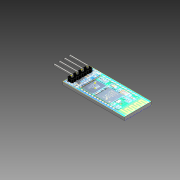
# Autodesk Inventor part: BLUTOOTH
Saved by Autodesk Inventor 2016 (Build 200138000, 138)
## iProperties
Created: 2017-05-25
Part Number: BLUTOOTH
Material: Generic
Document SubType Name: Modeling
Designer: USER
Density: 1 g/cm^3
Appearance: Default
Author: USER
Autodesk Inventor part; units mm, degrees
ref_plane "YZ Plane" through (0, 0, 0) normal (1, 0, 0) x (0, 1, 0)
ref_plane "XZ Plane" through (0, 0, 0) normal (0, 1, 0) x (-1, 0, 0)
ref_plane "XY Plane" through (0, 0, 0) normal (0, 0, 1) x (1, 0, 0)
sketch "Sketch1" plane through (0, 0, 0) normal (0, 0, 1) x (1, 0, 0)
  line L0 (-10.8819, 8.2952) -> (19.3441, 8.2952)
  line L1 (19.3441, 8.2952) -> (19.3441, -4.9318)
  line L2 (19.3441, -4.9318) -> (-10.8819, -4.9318)
  line L3 (-10.8819, -4.9318) -> (-10.8819, 8.2952)
  point P0 (0, 0)
  dimension "d0" = 30.226
  dimension "d1" = 13.227
  constraints: 8 end point, 1 parallel
  measures "d0" distance of L1.end L2.end
  measures "d1" distance of L0.end L1.end
extrude "Extrusion1" add sketch "Sketch1" along normal blind 1.5
sketch "Sketch2" plane through (0, 0, 1.5) normal (0, 0, 1) x (1, 0, 0)
  line L0 (-7.7625, -1.4726) -> (-7.7625, -3.0126)
  line L1 (-9.8024, 1.5674) -> (-8.2625, 1.5674)
  line L2 (-8.7125, 2.5174) -> (-9.3525, 2.5174)
  line L3 (-9.3525, 3.1574) -> (-8.7125, 3.1574)
  line L4 (-9.3525, 2.5174) -> (-9.3525, 3.1574)
  line L5 (-8.7125, 3.1574) -> (-8.7125, 2.5174)
  line L6 (-9.3525, 2.5174) -> (-8.7125, 3.1574) construction
  line L7 (-9.3525, 3.1574) -> (-8.7125, 2.5174) construction
  line L8 (-9.3524, 5.0573) -> (-9.3524, 5.6973)
  line L9 (-9.3524, 5.0573) -> (-8.7124, 5.6973) construction
  line L10 (-8.2625, 6.6474) -> (-9.8025, 6.6474)
  line L11 (-8.7124, 5.0573) -> (-9.3524, 5.0573)
  line L12 (-9.3524, 5.6973) -> (-8.7124, 5.6973)
  line L13 (-8.7124, 5.6973) -> (-8.7124, 5.0573)
  line L14 (-9.3524, 5.6973) -> (-8.7124, 5.0573) construction
  line L15 (-9.8025, 4.1074) -> (-8.2625, 4.1074)
  line L16 (-9.8025, -3.5126) -> (-8.2625, -3.5126)
  line L17 (-9.8024, -0.9726) -> (-8.2625, -0.9726)
  line L18 (-9.3524, -1.9227) -> (-8.7124, -1.9227)
  line L19 (-8.7124, -1.9227) -> (-8.7124, -2.5627)
  line L20 (-8.7124, -2.5627) -> (-9.3524, -2.5627)
  line L21 (-9.3524, -2.5627) -> (-9.3524, -1.9227)
  line L22 (-9.3525, 0.6174) -> (-8.7125, 0.6174)
  line L23 (-8.7125, 0.6174) -> (-8.7125, -0.0226)
  line L24 (-8.7125, -0.0226) -> (-9.3525, -0.0226)
  line L25 (-9.3525, -0.0226) -> (-9.3525, 0.6174)
  line L26 (-9.3525, 0.6174) -> (-8.7125, -0.0226) construction
  line L27 (-9.3524, -1.9227) -> (-8.7124, -2.5627) construction
  line L28 (-9.3524, -2.5627) -> (-8.7124, -1.9227) construction
  line L29 (-9.3525, -0.0226) -> (-8.7125, 0.6174) construction
  line L30 (-10.3025, 6.1474) -> (-10.3025, 4.6074)
  line L31 (-7.7625, 4.6074) -> (-7.7625, 6.1474)
  arc A0 (-7.7625, 6.1474) -> (-8.2625, 6.6474) centre (-8.2625, 6.1474) ccw
  arc A1 (-9.8025, 6.6474) -> (-10.3025, 6.1474) centre (-9.8025, 6.1474) ccw
  arc A2 (-8.2625, -3.5126) -> (-7.7625, -3.0126) centre (-8.2625, -3.0126) ccw
  arc A3 (-10.3025, -3.0126) -> (-9.8025, -3.5126) centre (-9.8025, -3.0126) ccw
  arc A4 (-8.2625, 4.1074) -> (-7.7625, 4.6074) centre (-8.2625, 4.6074) ccw
  arc A5 (-10.3025, 4.6074) -> (-9.8025, 4.1074) centre (-9.8025, 4.6074) ccw
  arc A6 (-7.7625, -1.4726) -> (-8.2625, -0.9726) centre (-8.2625, -1.4726) ccw
  line L32 (-10.3024, 2.0674) -> (-10.3023, 3.6074)
  line L33 (-9.8023, 4.1074) -> (-9.8025, 4.1074)
  arc A7 (-9.8023, 4.1074) -> (-10.3023, 3.6074) centre (-9.8023, 3.6074) ccw
  arc A8 (-10.3024, 2.0674) -> (-9.8024, 1.5674) centre (-9.8024, 2.0674) ccw
  line L34 (-9.8024, 1.5674) -> (-9.8024, 1.5674)
  line L35 (-10.3024, 1.0674) -> (-10.3024, -0.4726)
  line L36 (-7.7625, 2.0674) -> (-7.7625, 3.6074)
  line L37 (-8.2625, 4.1074) -> (-8.2625, 4.1074)
  arc A9 (-7.7625, 3.6074) -> (-8.2625, 4.1074) centre (-8.2625, 3.6074) ccw
  arc A10 (-8.2625, 1.5674) -> (-7.7625, 2.0674) centre (-8.2625, 2.0674) ccw
  arc A11 (-9.8024, 1.5674) -> (-10.3024, 1.0674) centre (-9.8024, 1.0674) ccw
  arc A12 (-10.3024, -0.4726) -> (-9.8024, -0.9726) centre (-9.8024, -0.4726) ccw
  line L38 (-8.2625, 1.5674) -> (-8.2625, 1.5674)
  line L39 (-7.7625, 1.0674) -> (-7.7625, -0.4726)
  line L40 (-8.2625, -0.9726) -> (-8.2625, -0.9726)
  line L41 (-9.8024, -0.9726) -> (-9.8024, -0.9726)
  line L42 (-10.3024, -1.4726) -> (-10.3024, -3.0237)
  arc A13 (-9.8024, -0.9726) -> (-10.3024, -1.4726) centre (-9.8024, -1.4726) ccw
  arc A14 (-8.2625, -0.9726) -> (-7.7625, -0.4726) centre (-8.2625, -0.4726) ccw
  arc A15 (-7.7625, 1.0674) -> (-8.2625, 1.5674) centre (-8.2625, 1.0674) ccw
  line L43 (-8.2625, -0.9726) -> (-9.8024, -0.9726)
  line L44 (-8.2625, 1.5674) -> (-9.8024, 1.5674)
  line L45 (-8.2625, 4.1074) -> (-9.8024, 4.1074)
  line L46 (-9.8024, -0.9726) -> (-8.2625, -0.9726)
  line L47 (-8.2625, -0.9726) -> (-9.8024, -0.9726)
  line L48 (-7.7625, -1.4726) -> (-7.7625, -3.0126)
  line L49 (-8.2625, -3.5126) -> (-9.8025, -3.5126)
  line L50 (-10.3024, -3.0237) -> (-10.3024, -1.4726)
  point P0 (-7.7625, 6.6911)
  dimension "d30" = 0.64
  dimension "d31" = 0.64
  dimension "d32" = 0.64
  dimension "d33" = 0.64
  dimension "d34" = 0.64
  dimension "d35" = 0.64
  dimension "d36" = 0.64
  dimension "d37" = 0.64
  dimension "d38" = 1.9001
  dimension "d39" = 1.9
  dimension "d40" = 1.9
  dimension "d41" = 0.5
  dimension "d42" = 0.5
  dimension "d43" = 0.5
  dimension "d44" = 0.5
  constraints: 102 end point, 45 point on circle, 35 tangent, 16 centre point, 12 equal radius, 12 parallel, 11 perpendicular, 6 point on line, 3 collinear, 3 horizontal
  measures "d30" distance of L18.end L19.end
  measures "d31" distance of L18.start L18.end
  measures "d32" distance of L22.end L24.start
  measures "d33" distance of L22.start L22.end
  measures "d34" distance of L3.end L2.start
  measures "d35" distance of L3.start L3.end
  measures "d36" distance of L9.end L11.start
  measures "d37" distance of L8.end L9.end
  measures "d38" distance between parallel lines of L24 L18
  measures "d39" distance between parallel lines of L2 L22
  measures "d40" distance between parallel lines of L11 L3
  measures "d41" radius of A0
  measures "d42" radius of A7
  measures "d43" radius of A9
  measures "d44" radius of A13
extrude "Extrusion2" add sketch "Sketch2" along normal blind 1.5 contours L17 A12 L35 A11 L1 A15 L39 A14 | L1 A8 L32 A7 L15 A9 L36 A10 | L15 A5 L30 A1 L10 A0 L31 A4 | L2 L4 L3 L5 | L8 L12 L13 L11 | L22 L23 L24 L25
extrude "Extrusion3" add sketch "Sketch2" along normal blind 1.5 contours L0 A2 L16 A3 L42 A13 L17 A6 | L18 L19 L20 L21
extrude "Extrusion4" add sketch "Sketch2" along normal blind 2.02 contours L2 L4 L3 L5 | L8 L12 L13 L11 | L18 L19 L20 L21 | L22 L23 L24 L25
ref_plane "Work Plane1" through (0, 0, 3.5) normal (0, 0, 1) x (1, 0, 0)
sketch "Sketch3" plane through (0, 0, 3.5) normal (0, 0, 1) x (1, 0, 0)
  line L0 (-8.7124, 5.0573) -> (-8.7124, 5.6973) projected
  line L1 (-8.7125, -0.0226) -> (-9.3525, -0.0226) projected
  line L2 (-9.3525, -0.0226) -> (-9.3525, 0.6174) projected
  line L3 (-9.3525, 0.6174) -> (-8.7125, 0.6174) projected
  line L4 (-8.7125, 0.6174) -> (-8.7125, -0.0226) projected
  line L5 (-9.3525, 3.1574) -> (-8.7125, 3.1574) projected
  line L6 (-8.7125, 3.1574) -> (-8.7125, 2.5174) projected
  line L7 (-8.7125, 2.5174) -> (-9.3525, 2.5174) projected
  line L8 (-9.3525, 2.5174) -> (-9.3525, 3.1574) projected
  line L9 (-8.7124, -1.9227) -> (-8.7124, -2.5627) projected
  line L10 (-8.7124, -2.5627) -> (-9.3524, -2.5627) projected
  line L11 (-9.3524, -2.5627) -> (-9.3524, -1.9227) projected
  line L12 (-9.3524, -1.9227) -> (-8.7124, -1.9227) projected
  line L13 (-9.3524, 5.6973) -> (-8.7124, 5.6973) projected
  line L14 (-8.7124, 5.6973) -> (-8.7124, 5.0573) projected
  line L15 (-8.7124, 5.0573) -> (-9.3524, 5.0573) projected
  line L16 (-9.3524, 5.0573) -> (-9.3524, 5.6973) projected
  arc A0 (-9.8024, 1.5674) -> (-10.3024, 1.0674) centre (-9.8024, 1.0674) ccw construction
  line L17 (-10.3024, 1.0674) -> (-10.3024, -0.4726) construction
  arc A1 (-10.3024, -0.4726) -> (-9.8024, -0.9726) centre (-9.8024, -0.4726) ccw construction
  arc A2 (-9.8024, -0.9726) -> (-10.3024, -1.4726) centre (-9.8024, -1.4726) ccw construction
  line L18 (-10.3024, -1.4726) -> (-10.3024, -3.0237) construction
  arc A3 (-10.3024, -3.0237) -> (-9.8025, -3.5126) centre (-9.8025, -3.0126) ccw construction
  line L19 (-9.8025, -3.5126) -> (-8.2625, -3.5126) construction
  arc A4 (-8.2625, -3.5126) -> (-7.7625, -3.0126) centre (-8.2625, -3.0126) ccw construction
  line L20 (-7.7625, -3.0126) -> (-7.7625, -1.4726) construction
  arc A5 (-7.7625, -1.4726) -> (-8.2625, -0.9726) centre (-8.2625, -1.4726) ccw construction
  arc A6 (-8.2625, -0.9726) -> (-7.7625, -0.4726) centre (-8.2625, -0.4726) ccw construction
  line L21 (-7.7625, -0.4726) -> (-7.7625, 1.0674) construction
  arc A7 (-7.7625, 1.0674) -> (-8.2625, 1.5674) centre (-8.2625, 1.0674) ccw construction
  arc A8 (-8.2625, 1.5674) -> (-7.7625, 2.0674) centre (-8.2625, 2.0674) ccw construction
  line L22 (-7.7625, 2.0674) -> (-7.7625, 3.6074) construction
  arc A9 (-7.7625, 3.6074) -> (-8.2625, 4.1074) centre (-8.2625, 3.6074) ccw construction
  arc A10 (-8.2625, 4.1074) -> (-7.7625, 4.6074) centre (-8.2625, 4.6074) ccw construction
  line L23 (-7.7625, 4.6074) -> (-7.7625, 6.1474) construction
  arc A11 (-7.7625, 6.1474) -> (-8.2625, 6.6474) centre (-8.2625, 6.1474) ccw construction
  line L24 (-8.2625, 6.6474) -> (-9.8025, 6.6474) construction
  arc A12 (-9.8025, 6.6474) -> (-10.3025, 6.1474) centre (-9.8025, 6.1474) ccw construction
  line L25 (-10.3025, 6.1474) -> (-10.3025, 4.6074) construction
  arc A13 (-10.3025, 4.6074) -> (-9.8024, 4.1074) centre (-9.8025, 4.6074) ccw construction
  arc A14 (-9.8024, 4.1074) -> (-10.3023, 3.6074) centre (-9.8023, 3.6074) ccw construction
  line L26 (-10.3023, 3.6074) -> (-10.3024, 2.0674) construction
  arc A15 (-10.3024, 2.0674) -> (-9.8024, 1.5674) centre (-9.8024, 2.0674) ccw construction
  line L27 (19.3441, 8.2952) -> (-10.8819, 8.2952) construction
  line L28 (-10.8819, 8.2952) -> (-10.8819, -4.9318) construction
  line L29 (-10.8819, -4.9318) -> (19.3441, -4.9318) construction
  line L30 (19.3441, -4.9318) -> (19.3441, 8.2952) construction
  arc A16 (-7.7625, -1.4726) -> (-8.2625, -0.9726) centre (-8.2625, -1.4726) ccw construction
  line L31 (-7.7625, -1.4726) -> (-7.7625, -3.0126) construction
  arc A17 (-8.2625, -3.5126) -> (-7.7625, -3.0126) centre (-8.2625, -3.0126) ccw construction
  line L32 (-8.2625, -3.5126) -> (-9.8025, -3.5126) construction
  arc A18 (-10.3024, -3.0237) -> (-9.8025, -3.5126) centre (-9.8025, -3.0126) ccw construction
  line L33 (-10.3024, -3.0237) -> (-10.3024, -1.4726) construction
  arc A19 (-9.8024, -0.9726) -> (-10.3024, -1.4726) centre (-9.8024, -1.4726) ccw construction
  arc A20 (-10.3024, -0.4726) -> (-9.8024, -0.9726) centre (-9.8024, -0.4726) ccw construction
  line L34 (-10.3024, -0.4726) -> (-10.3024, 1.0674) construction
  arc A21 (-9.8024, 1.5674) -> (-10.3024, 1.0674) centre (-9.8024, 1.0674) ccw construction
  arc A22 (-10.3024, 2.0674) -> (-9.8024, 1.5674) centre (-9.8024, 2.0674) ccw construction
  line L35 (-10.3024, 2.0674) -> (-10.3023, 3.6074) construction
  arc A23 (-9.8024, 4.1074) -> (-10.3023, 3.6074) centre (-9.8023, 3.6074) ccw construction
  arc A24 (-10.3025, 4.6074) -> (-9.8024, 4.1074) centre (-9.8025, 4.6074) ccw construction
  line L36 (-10.3025, 4.6074) -> (-10.3025, 6.1474) construction
  arc A25 (-9.8025, 6.6474) -> (-10.3025, 6.1474) centre (-9.8025, 6.1474) ccw construction
  line L37 (-9.8025, 6.6474) -> (-8.2625, 6.6474) construction
  arc A26 (-7.7625, 6.1474) -> (-8.2625, 6.6474) centre (-8.2625, 6.1474) ccw construction
  line L38 (-7.7625, 6.1474) -> (-7.7625, 4.6074) construction
  arc A27 (-8.2625, 4.1074) -> (-7.7625, 4.6074) centre (-8.2625, 4.6074) ccw construction
  arc A28 (-7.7625, 3.6074) -> (-8.2625, 4.1074) centre (-8.2625, 3.6074) ccw construction
  line L39 (-7.7625, 3.6074) -> (-7.7625, 2.0674) construction
  arc A29 (-8.2625, 1.5674) -> (-7.7625, 2.0674) centre (-8.2625, 2.0674) ccw construction
  arc A30 (-7.7625, 1.0674) -> (-8.2625, 1.5674) centre (-8.2625, 1.0674) ccw construction
  line L40 (-7.7625, 1.0674) -> (-7.7625, -0.4726) construction
  arc A31 (-8.2625, -0.9726) -> (-7.7625, -0.4726) centre (-8.2625, -0.4726) ccw construction
  point P0 (0, 0)
ref_plane "Work Plane2" through (-17.8819, -4.9318, 0) normal (-1, 0, 0) x (0, 0, 1)
sketch "Sketch4" plane through (-17.8819, -4.9318, 0) normal (-1, 0, 0) x (0, 0, 1)
  line L0 (3.5011, 3.0104) -> (4.1411, 3.0104)
  line L1 (3.5011, 3.0104) -> (4.1411, 2.3704) construction
  line L2 (4.1411, 3.0104) -> (4.1411, 2.3704)
  line L3 (4.1411, 2.3704) -> (3.5011, 2.3704)
  line L4 (3.5011, 2.3704) -> (3.5011, 3.0104)
  line L5 (3.5011, 2.3704) -> (4.1411, 3.0104) construction
  line L6 (4.1411, 7.4505) -> (3.5011, 7.4505)
  line L7 (3.5011, 8.0905) -> (4.1411, 8.0905)
  line L8 (4.1411, 8.0905) -> (4.1411, 7.4505)
  line L9 (3.5011, 7.4505) -> (4.1411, 8.0905) construction
  line L10 (3.5011, 8.0905) -> (4.1411, 7.4505) construction
  line L11 (3.5011, 7.4505) -> (3.5011, 8.0905)
  line L12 (3.5012, 9.9904) -> (3.5012, 10.6304)
  line L13 (3.5012, 9.9904) -> (4.1412, 10.6304) construction
  line L14 (4.1412, 9.9904) -> (3.5012, 9.9904)
  line L15 (4.1412, 10.6304) -> (4.1412, 9.9904)
  line L16 (3.5012, 10.6304) -> (4.1412, 9.9904) construction
  line L17 (3.5012, 10.6304) -> (4.1412, 10.6304)
  line L18 (4.1411, 4.9105) -> (3.5011, 4.9105)
  line L19 (3.5011, 5.5505) -> (4.1411, 5.5505)
  line L20 (4.1411, 5.5505) -> (4.1411, 4.9105)
  line L21 (3.5011, 4.9105) -> (3.5011, 5.5505)
  line L22 (3.5011, 5.5505) -> (4.1411, 4.9105) construction
  line L23 (3.5011, 4.9105) -> (4.1411, 5.5505) construction
  line L24 (2.4101, 9.0392) -> (2.41, 9.0392)
  line L25 (2.4101, 6.4992) -> (2.4101, 6.4992)
  line L26 (2.4101, 3.9592) -> (2.4101, 3.9592)
  point P0 (0, 4.9318)
  point P1 (2.2355, 10.9967)
  point P2 (2.2355, 1.8367)
  point P3 (2.2355, 9.4567)
  point P4 (2.2356, 8.4567)
  point P5 (2.2356, 6.9167)
  point P6 (2.2356, 5.9167)
  point P7 (2.2356, 3.8767)
  point P8 (2.2356, 4.3767)
  point P9 (2.2356, 3.3767)
  point P10 (2.2356, 3.8767)
  point P11 (2.2356, 8.9567)
  dimension "d53" = 0.64
  dimension "d54" = 0.64
  dimension "d55" = 0.64
  dimension "d56" = 0.64
  dimension "d57" = 0.64
  dimension "d58" = 0.64
  dimension "d59" = 0.64
  dimension "d60" = 0.64
  dimension "d61" = 1.9001
  dimension "d62" = 1.9
  dimension "d63" = 1.9
  constraints: 54 end point, 8 parallel, 5 perpendicular, 2 horizontal, 1 point on line
  measures "d53" distance of L2.start L2.end
  measures "d54" distance of L1.start L2.start
  measures "d55" distance of L19.end L18.start
  measures "d56" distance of L19.start L19.end
  measures "d57" distance of L7.end L6.start
  measures "d58" distance of L11.end L7.end
  measures "d59" distance of L15.start L15.end
  measures "d60" distance of L12.end L15.start
  measures "d61" distance between parallel lines of L18 L0
  measures "d62" distance between parallel lines of L6 L19
  measures "d63" distance between parallel lines of L14 L7
ref_plane "Work Plane4" through (-17.8819, 3.1587, 3.8211) normal (0, 0, 1) x (1, 0, 0)
ref_plane "Work Plane5" through (-9.0325, 0.6174, 3.52) normal (1, 0, 0) x (0, 1, 0)
sketch "Sketch5" plane through (-17.8819, 3.1587, 3.8211) normal (0, 0, 1) x (1, 0, 0)
  line L0 (0, -5.0801) -> (0, -5.7201) projected
  line L1 (0, -2.54) -> (0, -3.18) projected
  line L2 (0, 0) -> (0, -0.64) projected
  line L3 (0, 2.5399) -> (0, 1.8999) projected
  point P0 (17.8819, -3.1587)
sketch "Sketch6" plane through (-9.0325, 0.6174, 3.52) normal (1, 0, 0) x (0, 1, 0)
  point P0 (-0.6174, -3.52)
sketch "Sketch7" plane through (-17.8819, 3.1587, 3.8211) normal (0, 0, 1) x (1, 0, 0)
  line L0 (8.5294, -5.7213) -> (8.5294, -5.0813) projected
  line L1 (8.5294, -3.1813) -> (8.5294, -2.5413) projected
  line L2 (8.5294, -0.6413) -> (8.5294, -0.0013) projected
  line L3 (8.5295, 1.8987) -> (8.5295, 2.5387) projected
  point P0 (17.8819, -3.1587)
sketch "Sketch8" plane through (-9.0325, 0.6174, 3.52) normal (1, 0, 0) x (0, 1, 0)
  line L0 (-3.1801, 0.3011) -> (-2.5401, 0.3011) projected
  line L1 (-0.64, 0.3011) -> (0, 0.3011) projected
  line L2 (1.9, 0.3011) -> (2.54, 0.3011) projected
  line L3 (4.44, 0.3011) -> (5.08, 0.3011) projected
  point P0 (-0.6174, -3.52)
sketch "Sketch9" plane through (-17.8819, 3.1587, 3.8211) normal (0, 0, 1) x (1, 0, 0)
  line L0 (0, -5.4007) -> (8.8472, -5.4007)
  line L1 (8.8472, -2.8613) -> (0, -2.8613)
  line L2 (8.8472, -0.3213) -> (0, -0.3213)
  line L3 (8.8472, 2.2187) -> (0, 2.2187)
  point P0 (17.8819, -3.1587)
  constraints: 8 end point, 4 horizontal
sketch "Sketch10" plane through (-9.0325, 0.6174, 3.52) normal (1, 0, 0) x (0, 1, 0)
  line L0 (-0.32, 0.3312) -> (-0.32, 0)
  line L1 (0, 0) -> (-0.64, 0) projected
  line L2 (1.9, 0) -> (2.54, 0) projected
  line L3 (2.22, 0) -> (2.22, 0.3312)
  line L4 (4.44, 0) -> (5.08, 0) projected
  line L5 (4.76, 0) -> (4.76, 0.3312)
  point P0 (-0.6174, -3.52)
  constraints: 6 end point, 3 midpoint, 2 vertical
extrude "Extrusion5" add sketch "Sketch4" against normal blind 9.169
fillet "Fillet1" radius 0.3 1 edges at (-9.3524, 5.378, 3.5012)
fillet "Fillet2" radius 0.3 1 edges at (-9.3525, 2.838, 3.5011)
fillet "Fillet3" radius 0.3 1 edges at (-9.3525, 0.298, 3.5011)
fillet "Fillet4" radius 0.3 1 edges at (-9.3524, -2.2421, 3.5011)
fillet "Fillet5" radius 0.3 4 edges at (-8.7129, 5.3786, 4.1412) (-8.7129, 2.8387, 4.1411) (-8.7129, 0.2987, 4.1411) (-8.7129, -2.2414, 4.1411)
sketch "Sketch11" plane through (0, 0, 1.5) normal (0, 0, 1) x (1, 0, 0)
  line L0 (-10.8815, 8.2937) -> (19.2548, 8.2937) construction
  line L1 (19.2548, 8.2937) -> (19.2548, -4.9334) construction
  line L2 (19.2548, -4.9334) -> (-10.8815, -4.9334) construction
  line L3 (-10.8815, -4.9334) -> (-10.8815, 8.2937) construction
  point P0 (0, 0)
  constraints: 2 other
sketch "Sketch12" plane through (0, 0, 0) normal (0, 0, -1) x (-1, 0, 0)
  line L0 (10.8819, 8.2952) -> (-19.3441, 8.2952) projected
  line L1 (-19.3441, 8.2952) -> (10.8819, 8.2952) construction
  line L2 (10.8819, 8.2952) -> (10.8819, -4.5926) construction
  line L3 (10.8819, -4.5926) -> (-19.3441, -4.5926) construction
  line L4 (-19.3441, -4.5926) -> (-19.3441, 8.2952) construction
  point P0 (0, 0)
  constraints: 1 coincident, 2 other
ref_plane "Work Plane3" through (-17.8819, 3.1587, 4.1411) normal (0, 0, 1) x (1, 0, 0)
body "Solid1"
